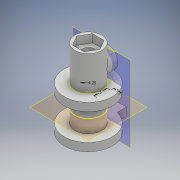
# Autodesk Inventor part: stationarySpindle
Saved by Autodesk Inventor 2018 (Build 220112000, 112)
## iProperties
Created: 2018-11-25
Part Number: stationarySpindle
Material: Generic
Document SubType Name: Modeling
Designer: Prakash
Density: 1 g/cm^3
Appearance: Default
Author: Prakash
Autodesk Inventor part; units mm, degrees
ref_plane "YZ Plane" through (0, 0, 0) normal (1, 0, 0) x (0, 1, 0)
ref_plane "XZ Plane" through (0, 0, 0) normal (0, 1, 0) x (-1, 0, 0)
ref_plane "XY Plane" through (0, 0, 0) normal (0, 0, 1) x (1, 0, 0)
sketch "Sketch1" plane through (0, 0, 0) normal (0, 0, 1) x (1, 0, 0)
  circle A0 centre (0, 0) radius 5
  circle A1 centre (0, 0) radius 9
  circle A2 centre (0, 0) radius 2.125
  dimension "d0" = 10
  dimension "d1" = 18
  dimension "d2" = 4.25
  constraints: 3 centre point, 3 coincident
  measures "d0" diameter of A0
  measures "d1" diameter of A1
  measures "d2" diameter of A2
extrude "Extrusion1" add sketch "Sketch1" against normal blind 10 contours A0 | A2
extrude "Extrusion2" add sketch "Sketch1" along normal blind 3 contours A0 | A1 | A2
sketch "Sketch2" plane through (0, 0, -10) normal (0, 0, -1) x (-1, 0, 0)
  circle A0 centre (0, 0) radius 9 projected
extrude "Extrusion3" add sketch "Sketch2" along normal blind 3
sketch "Sketch3" plane through (0, 0, 3) normal (0, 0, 1) x (1, 0, 0)
  circle A0 centre (0, 0) radius 5 projected
  circle A1 centre (0, 0) radius 2.125
  dimension "d9" = 4.25
  constraints: 1 centre point, 1 coincident
  measures "d9" diameter of A1
extrude "Extrusion4" add sketch "Sketch3" along normal blind 10
ref_plane "Work Plane1" through (0, 0, -5) normal (0, 0, 1) x (1, 0, 0)
sketch "Sketch4" plane through (0, 0, -5) normal (0, 0, 1) x (1, 0, 0)
  circle A0 centre (0, 0) radius 5 projected
  arc A1 (1.5, 4.7697) -> (-1.5, 4.7697) centre (0, 0) ccw
  line L0 (0, 0) -> (0, 5) construction
  line L1 (-1.5, 4.7697) -> (-1.5, 9.7697)
  line L2 (-1.5, 9.7697) -> (1.5, 9.7697)
  line L3 (1.5, 9.7697) -> (1.5, 4.7697)
  dimension "d12" = 5
  dimension "d13" = 3
  constraints: 8 end point, 5 point on circle, 3 vertical, 1 centre point, 1 concentric, 1 perpendicular, 1 other
  measures "d12" distance of L1.start L1.end
  measures "d13" distance of L1.end L2.end
ref_plane "Work Plane2" through (0, 5, 2) normal (0, 1, 0) x (-1, 0, 0)
sketch "Sketch5" plane through (0, 5, 2) normal (0, 1, 0) x (-1, 0, 0)
  line L0 (5, 11) -> (-5, 11) projected
  line L1 (-5, 1) -> (5, 1) projected
  line L2 (-5, 11) -> (5, 1) construction
  line L3 (5, 11) -> (-5, 1) construction
  point P0 (0, -2)
  point P1 (0, 6)
  constraints: 4 end point, 1 midpoint, 1 perpendicular
extrude "Extrusion6" cut sketch "Sketch3" against normal up to surface (16 mm away) contours A1
sketch "Sketch6" plane through (0, 5, 2) normal (0, 1, 0) x (-1, 0, 0)
  line L0 (5, 11) -> (-5, 1) construction
  line L1 (-5, 11) -> (5, 1) construction
  circle A0 centre (0, 6) radius 4
  point P0 (0, -2)
  dimension "d18" = 8
  constraints: 1 centre point, 1 coincident
  measures "d18" diameter of A0
extrude "Extrusion7" add sketch "Sketch6" against normal up to surface
extrude "Extrusion8" add sketch "Sketch6" along normal blind 2.125
sketch "Sketch7" plane through (0, 7.125, 8) normal (0, 1, 0) x (1, 0, 0)
  line L0 (5, -5) -> (-5, 5) construction
  line L1 (-5, -5) -> (5, 5) construction
  circle A0 centre (0, 0) radius 4 projected
  circle A1 centre (0, 0) radius 2.5275
  point P0 (0, 8)
  dimension "d23" = 5.055
  constraints: 1 centre point, 1 coincident
  measures "d23" diameter of A1
extrude "Extrusion9" cut sketch "Sketch7" against normal blind 3.81 contours A1
sketch "Sketch8" plane through (0, 7.125, 8) normal (0, 1, 0) x (1, 0, 0)
  line L0 (-5, -5) -> (5, 5) construction
  line L1 (5, -5) -> (-5, 5) construction
  circle A0 centre (0, 0) radius 2.6545
  point P0 (0, 8)
  dimension "d26" = 5.309
  constraints: 1 centre point, 1 coincident
  measures "d26" diameter of A0
loft "Loft1" cut profiles "Sketch8" section 1 edges at (-2.5275, 3.315, 8)
sketch "Sketch9" plane through (0, 3.315, 8) normal (0, 1, 0) x (1, 0, 0)
  line L0 (-5, -5) -> (5, 5) construction
  line L1 (5, -5) -> (-5, 5) construction
  circle A0 centre (0, 0) radius 1.8
  point P0 (0, 8)
  dimension "d31" = 3.6
  constraints: 1 centre point, 1 coincident
  measures "d31" diameter of A0
extrude "Extrusion10" cut sketch "Sketch9" against normal up to surface
sketch "Sketch10" plane through (0, 0, -13) normal (0, 0, -1) x (-1, 0, 0)
  circle A0 centre (0, 0) radius 2.125 projected
  circle A1 centre (0, 0) radius 9 projected
  line L0 (0, 0) -> (0, 9) construction
  line L1 (-2, 8.775) -> (-2, 12.275)
  line L2 (-2, 12.275) -> (2, 12.275)
  line L3 (2, 12.275) -> (2, 8.775)
  arc A2 (2, 8.775) -> (-2, 8.775) centre (0, 0) ccw
  dimension "d34" = 3.5
  dimension "d35" = 4
  constraints: 8 end point, 6 point on circle, 2 perpendicular, 2 vertical, 1 centre point, 1 other
  measures "d34" distance of L1.start L1.end
  measures "d35" distance of L1.end L2.end
extrude "Extrusion11" add sketch "Sketch10" against normal up to surface (3 mm away) contours A1 L1 L2 L3
sketch "Sketch12" plane through (0, 0, 13) normal (0, 0, 1) x (1, 0, 0)
  line L0 (2.1651, -3.75) -> (-2.1651, -3.75)
  line L1 (-2.1651, -3.75) -> (-4.3301, 0)
  line L2 (-4.3301, 0) -> (-2.1651, 3.75)
  line L3 (-2.1651, 3.75) -> (2.1651, 3.75)
  line L4 (2.1651, 3.75) -> (4.3301, 0)
  line L5 (4.3301, 0) -> (2.1651, -3.75)
  circle A0 centre (0, 0) radius 5 projected
  line L6 (0, 0) -> (0, -5) construction
  circle A1 centre (0, 0) radius 5
  point P0 (0, 5)
  dimension "d39" = 7.5
  constraints: 14 end point, 2 coincident, 1 horizontal, 1 point on circle, 1 vertical, 1 vertical alignment, 15 other
  measures "d39" distance between parallel lines of L0 L3
extrude "Extrusion12" add sketch "Sketch12" along normal blind 3
body "Solid1"
